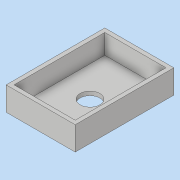
# Autodesk Inventor part: тело
Saved by Autodesk Inventor 2019 (Build 230136000, 136)
## iProperties
Created: 2019-09-06
Part Number: тело
Material: Типовые
Document SubType Name: Modeling
Designer: Iliga
Density: 1 g/cm^3
Appearance: По умолчанию
Mass: 236.83 g
Surface Area: 2382.33 cm^2
Volume: 236.83 cm^3
Author: Iliga
Autodesk Inventor part; units mm, degrees
ref_plane "РабПлоскость1" through (0, -35, 0) normal (0, 1, 0) x (-1, 0, 0)
ref_plane "РабПлоскость25" through (100, -155, 0) normal (-1, 0, 0) x (0, 0, 1)
ref_plane "РабПлоскость26" through (84, -165, -19) normal (-1, 0, 0) x (0, 0, 1)
sketch "Эскиз130" plane through (0, 0, 0) normal (0, 1, 0) x (-1, 0, 0)
  line L0 (-17.5, 25) -> (17.5, 25)
  line L1 (17.5, 25) -> (17.5, -25)
  line L2 (17.5, -25) -> (-17.5, -25)
  line L3 (-17.5, -25) -> (-17.5, 25)
  line L4 (-17.5, 25) -> (17.5, -25) construction
  line L5 (17.5, 25) -> (-17.5, -25) construction
  point P0 (0, 0)
  dimension "d710" = 50
  dimension "d711" = 35
  constraints: 12 end point, 2 midpoint, 2 parallel, 1 horizontal, 1 perpendicular
  measures "d710" distance of L0.end L1.end
  measures "d711" distance of L1.end L2.end
extrude "Выдавливание115" add sketch "Эскиз130" along normal blind 2
sketch "Эскиз131" plane through (0, 2, 0) normal (0, 1, 0) x (1, 0, 0)
  line L0 (15.5, -23) -> (-15.5, -23)
  line L1 (-15.5, -23) -> (-15.5, 23)
  line L2 (-15.5, 23) -> (15.5, 23)
  line L3 (15.5, 23) -> (15.5, -23)
  line L4 (15.5, -23) -> (-15.5, 23) construction
  line L5 (-15.5, -23) -> (15.5, 23) construction
  line L6 (-17.5, 25) -> (-17.5, -25) projected
  line L7 (17.5, 25) -> (-17.5, 25) projected
  line L8 (-17.5, -25) -> (17.5, -25) projected
  line L9 (17.5, -25) -> (17.5, 25) projected
  line L10 (-17.5, -25) -> (17.5, -25) projected
  line L11 (17.5, -25) -> (17.5, 25) projected
  line L12 (17.5, 25) -> (-17.5, 25) projected
  line L13 (-17.5, 25) -> (-17.5, -25) projected
  point P0 (0, 0)
  dimension "d714" = 2
  dimension "d715" = 2
  constraints: 12 end point, 2 midpoint, 2 parallel, 1 horizontal, 1 perpendicular
  measures "d714" distance between parallel lines of L1 L6
  measures "d715" distance between parallel lines of L7 L2
extrude "Выдавливание116" add sketch "Эскиз131" along normal blind 10
sketch "Эскиз132" plane through (0, 2, 0) normal (0, 1, 0) x (1, 0, 0)
  circle A0 centre (0, 0) radius 5
  dimension "d718" = 10
  dimension "d12" = 100
  dimension "d14" = 17
  dimension "d26" = 5
  constraints: 1 centre point, 1 coincident
  measures "d718" diameter of A0
extrude "Выдавливание117" cut sketch "Эскиз132" against normal blind 10
sketch "Эскиз6" plane through (0, -35, -85) normal (0, -1, 0) x (1, 0, 0)
  arc A0 (29.3991, 164.4544) -> (0, 170) centre (-5, 62.7941) ccw projected
  line L0 (0, 170) -> (0, 0) projected
  arc A1 (0, 0) -> (29.3991, 5.5456) centre (-5, 107.2059) ccw projected
  arc A2 (29.3991, 5.5456) -> (100, 85) centre (-5, 107.2059) ccw projected
  arc A3 (100, 85) -> (29.3991, 164.4544) centre (-5, 62.7941) ccw projected
  point P0 (0, 85)
  constraints: 4 end point, 1 horizontal, 1 point on circle, 1 vertical
sketch "Эскиз114" plane through (2, -165, 82.8837) normal (1, 0, 0) x (0, 0, -1)
  circle A0 centre (120.1897, 5) radius 1
  line L0 (-2.1163, 0) -> (167.8837, 0) construction
  line L1 (82.8837, 0) -> (82.8837, 60.2174) construction
  circle A1 centre (45.5777, 5) radius 1
  point P0 (82.8837, 165)
  dimension "d609" = 2
  dimension "d610" = 37.306
  dimension "d611" = 5
  constraints: 2 centre point, 2 end point, 1 midpoint, 1 symmetric about line, 1 vertical, 1 other
  measures "d609" diameter of A0
  measures "d610" distance from line of L1 A0.centre
  measures "d611" distance from line of L0 A0.centre
sketch "Эскиз115" plane through (2, -165, 82.8837) normal (1, 0, 0) x (0, 0, -1)
  line L0 (167.7717, 0) -> (0, 0) construction
  line L1 (82.8837, 130) -> (82.8837, 0) construction
  line L2 (63.8837, 0) -> (101.8837, 0)
  line L3 (101.8837, 0) -> (101.8837, 20)
  line L4 (101.8837, 20) -> (63.8837, 20)
  line L5 (63.8837, 20) -> (63.8837, 0)
  line L6 (65.8837, 2) -> (99.8837, 2)
  line L7 (99.8837, 2) -> (99.8837, 18)
  line L8 (99.8837, 18) -> (65.8837, 18)
  line L9 (65.8837, 18) -> (65.8837, 2)
  line L10 (65.8837, 2) -> (99.8837, 18) construction
  line L11 (99.8837, 2) -> (65.8837, 18) construction
  point P0 (82.8837, 165)
  point P1 (145.8837, 0)
  point P2 (82.8837, 20)
  point P3 (82.8837, 10)
  dimension "d614" = 38
  dimension "d615" = 20
  dimension "d616" = 2
  dimension "d617" = 2
  dimension "d618" = 2
  constraints: 20 end point, 4 parallel, 3 midpoint, 3 point on line, 2 horizontal, 2 perpendicular
  measures "d614" distance between parallel lines of L5 L3
  measures "d615" distance between parallel lines of L4 L0
  measures "d616" distance between parallel lines of L0 L6
  measures "d617" distance between parallel lines of L3 L7
  measures "d618" distance between parallel lines of L4 L8
sketch "Эскиз116" plane through (0, -165, -85) normal (0, -1, 0) x (1, 0, 0)
  arc A0 (91.9272, 104) -> (2, 167.8837) centre (-5, 62.7941) ccw construction
  arc A1 (97.9549, 85) -> (92.7533, 102) centre (-5, 62.7941) ccw construction
  arc A2 (97.9549, 85) -> (91.9272, 104) centre (-5, 62.7941) ccw construction
  arc A3 (91.9272, 66) -> (97.9549, 85) centre (-5, 107.206) ccw
  line L0 (2, 66) -> (100.2736, 66) construction
  arc A4 (100.2736, 66) -> (97.9549, 85) centre (-5, 62.7941) ccw projected
  line L1 (91.9272, 66) -> (100.2736, 66)
  point P0 (0, 85)
  point P1 (36.5, 159.5958)
  dimension "d621" = 22.206
  constraints: 2 end point, 2 point on circle, 1 centre point, 1 collinear, 1 point on line, 1 vertical alignment
  measures "d621" vertical distance of A3.centre point (0, 85)
sketch "Эскиз117" plane through (2, -165, 82.8837) normal (1, 0, 0) x (0, 0, -1)
  line L0 (101.8837, 20) -> (101.8837, 0) projected
  line L1 (63.8837, 20) -> (101.8837, 20) projected
  line L2 (63.8837, 0) -> (63.8837, 20) projected
  line L3 (63.8837, 0) -> (101.8837, 0)
  point P0 (82.8837, 165)
  constraints: 2 end point, 1 horizontal
sketch "Эскиз118" plane through (0, -165, -85) normal (0, -1, 0) x (1, 0, 0)
  line L0 (2, 66) -> (2, 104) projected
  line L1 (2, 66) -> (91.9272, 66) projected
  arc A0 (91.9272, 66) -> (97.9549, 85) centre (-5, 107.206) ccw projected
  line L2 (97.9549, 85) -> (100, 85) projected
  arc A1 (100, 85) -> (94.0968, 104) centre (-5, 62.7941) ccw projected
  line L3 (2, 104) -> (94.0968, 104) projected
  line L4 (2, 104) -> (4, 104)
  line L5 (4, 104) -> (4, 66)
  line L6 (4, 66) -> (2, 66)
  line L7 (2, 66) -> (2, 104)
  point P0 (0, 85)
  dimension "d626" = 2
  constraints: 8 end point, 2 parallel, 1 horizontal, 1 perpendicular, 1 point on line
  measures "d626" distance between parallel lines of L5 L0
sketch "Эскиз119" plane through (0, -165, -85) normal (0, -1, 0) x (1, 0, 0)
  arc A0 (100, 85) -> (94.0968, 104) centre (-5, 62.7941) ccw construction
  line L0 (4, 104) -> (4, 66) construction
  line L1 (4, 85) -> (65.3021, 85) construction
  arc A1 (94.0968, 66) -> (100, 85) centre (-5, 107.2059) ccw
  arc A2 (91.9272, 66) -> (97.9549, 85) centre (-5, 107.206) ccw construction
  line L2 (100, 85) -> (97.9549, 85)
  line L3 (94.0968, 66) -> (91.9272, 66)
  arc A3 (91.9272, 66) -> (97.9549, 85) centre (-5, 107.206) ccw
  point P0 (0, 85)
  constraints: 6 end point, 4 point on circle, 2 centre point, 2 horizontal, 2 symmetric about line, 1 coincident, 1 midpoint, 1 parallel, 1 point on line, 1 other
sketch "Эскиз120" plane through (4, -147, 17) normal (0, -1, 0) x (1, 0, 0)
  line L0 (0, 0) -> (2, 0)
  line L1 (2, 0) -> (2, -34)
  line L2 (2, -34) -> (0, -34)
  line L3 (0, -34) -> (0, 0)
  point P0 (-4, -17)
  dimension "d631" = 2
  constraints: 8 end point, 2 parallel, 1 coincident, 1 horizontal, 1 perpendicular
  measures "d631" distance between parallel lines of L3 L1
sketch "Эскиз121" plane through (0, 0, 0) normal (1, 0, 0) x (0, 1, 0)
  line L0 (-145, -19) -> (-145, 19) construction
  line L1 (-165, -19) -> (-145, -19) construction
  line L2 (-165, 19) -> (-165, -19) construction
  line L3 (-145, 19) -> (-165, 19) construction
  line L4 (-158, -19) -> (-152, -19)
  line L5 (-152, -19) -> (-152, -25)
  line L6 (-152, -25) -> (-158, -25)
  line L7 (-158, -25) -> (-158, -19)
  circle A0 centre (-155, -22) radius 1
  line L8 (-158, 25) -> (-152, 25)
  line L9 (-152, 25) -> (-152, 19)
  line L10 (-152, 19) -> (-158, 19)
  line L11 (-158, 19) -> (-158, 25)
  circle A1 centre (-155, 22) radius 1
  line L12 (-155, 19) -> (-155, -19) construction
  point P0 (0, 0)
  dimension "d634" = 6
  dimension "d635" = 6
  dimension "d636" = 2
  dimension "d637" = 3
  dimension "d638" = 3
  dimension "d639" = 6
  dimension "d640" = 6
  dimension "d641" = 2
  dimension "d642" = 3
  dimension "d643" = 3
  constraints: 18 end point, 4 midpoint, 4 parallel, 2 centre point, 2 horizontal, 2 perpendicular
  measures "d634" distance of L5.end L6.end
  measures "d635" distance of L4.end L5.end
  measures "d636" diameter of A0
  measures "d637" distance from line of L6 A0.centre
  measures "d638" distance from line of L7 A0.centre
  measures "d639" distance of L9.end L10.end
  measures "d640" distance of L8.end L9.end
  measures "d641" diameter of A1
  measures "d642" distance from line of L10 A1.centre
  measures "d643" distance from line of L11 A1.centre
sketch "Эскиз122" plane through (0, -158, 19) normal (0, -1, 0) x (1, 0, 0)
  line L0 (0, 0) -> (0, 6) projected
  line L1 (0, 0) -> (4, 0) projected
  line L2 (6, 0) -> (4, 0) projected
  line L3 (6, 6) -> (6, 0) projected
  line L4 (0, 6) -> (6, 6) projected
  line L5 (0, -44) -> (0, -38) projected
  line L6 (0, -44) -> (6, -44) projected
  line L7 (6, -38) -> (6, -44) projected
  line L8 (4, -38) -> (6, -38) projected
  line L9 (0, -38) -> (4, -38) projected
  line L10 (0, 6) -> (4, 6)
  line L11 (4, 6) -> (4, -44)
  line L12 (4, -44) -> (0, -44)
  line L13 (0, -44) -> (0, 6)
  line L14 (0, -44) -> (6, -44) projected
  point P0 (0, -19)
  dimension "d646" = 4
  constraints: 8 end point, 2 parallel, 1 horizontal, 1 perpendicular, 1 point on line
  measures "d646" distance between parallel lines of L11 L13
sketch "Эскиз123" plane through (0, -165, -85) normal (0, -1, 0) x (1, 0, 0)
  line L0 (32, 66) -> (34, 66)
  line L1 (34, 66) -> (34, 63)
  line L2 (34, 63) -> (32, 63)
  line L3 (32, 63) -> (32, 66)
  line L4 (4, 104) -> (4, 66) projected
  line L5 (94.0968, 66) -> (4, 66) projected
  line L6 (32, 107) -> (34, 107)
  line L7 (34, 107) -> (34, 104)
  line L8 (34, 104) -> (32, 104)
  line L9 (32, 104) -> (32, 107)
  line L10 (4, 104) -> (94.0968, 104) projected
  line L11 (36.5, 107) -> (38.5, 107)
  line L12 (38.5, 107) -> (38.5, 104)
  line L13 (38.5, 104) -> (36.5, 104)
  line L14 (36.5, 104) -> (36.5, 107)
  line L15 (36.5, 66) -> (38.5, 66)
  line L16 (38.5, 66) -> (38.5, 63)
  line L17 (38.5, 63) -> (36.5, 63)
  line L18 (36.5, 63) -> (36.5, 66)
  point P0 (0, 85)
  dimension "d650" = 30
  dimension "d651" = 2
  dimension "d652" = 3
  dimension "d653" = 2
  dimension "d654" = 3
  dimension "d655" = 2
  dimension "d656" = 3
  dimension "d657" = 2
  dimension "d658" = 3
  dimension "d659" = 30
  dimension "d660" = 2.5
  dimension "d661" = 2.5
  constraints: 32 end point, 8 parallel, 4 horizontal, 4 perpendicular, 4 point on line
  measures "d650" distance between parallel lines of L4 L1
  measures "d651" distance between parallel lines of L1 L3
  measures "d652" distance of L0.end L1.end
  measures "d653" distance between parallel lines of L7 L9
  measures "d654" distance of L6.end L7.end
  measures "d655" distance between parallel lines of L12 L14
  measures "d656" distance of L11.end L12.end
  measures "d657" distance between parallel lines of L16 L18
  measures "d658" distance of L15.end L16.end
  measures "d659" distance between parallel lines of L4 L7
  measures "d660" distance between parallel lines of L14 L7
  measures "d661" distance between parallel lines of L18 L1
sketch "Эскиз124" plane through (36.5, -145, -19) normal (0, 0, 1) x (1, 0, 0)
  line L0 (0, 0) -> (2, 0) projected
  line L1 (2, 0) -> (2, 2) projected
  line L2 (0, 2) -> (2, 2) projected
  line L3 (0, 0) -> (0, 2) projected
  line L4 (-4.5, 0) -> (-2.5, 0) projected
  line L5 (-2.5, 0) -> (-2.5, 2) projected
  line L6 (-4.5, 2) -> (-2.5, 2) projected
  line L7 (-4.5, 0) -> (-4.5, 2) projected
  point P0 (-36.5, 145)
  dimension "d667" = 2
  dimension "d668" = 9.5
  dimension "d669" = 10
  constraints: 2 centre point, 2 end point, 1 symmetric about line, 1 vertical, 1 other
sketch "Эскиз126" plane through (0, -165, -85) normal (0, -1, 0) x (1, 0, 0)
  circle A0 centre (16, 79) radius 1
  circle A1 centre (16, 91) radius 1
  line L0 (4, 104) -> (4, 66) projected
  line L1 (4, 85) -> (100.0263, 85) construction
  circle A2 centre (31, 79) radius 1
  circle A3 centre (31, 91) radius 1
  circle A4 centre (71, 75) radius 1
  circle A5 centre (71, 95) radius 1
  point P0 (0, 85)
  dimension "d674" = 2
  dimension "d675" = 2
  dimension "d676" = 12
  dimension "d677" = 12
  dimension "d678" = 6
  dimension "d679" = 2
  dimension "d680" = 2
  dimension "d681" = 12
  dimension "d683" = 27
  dimension "d684" = 6
  dimension "d685" = 2
  dimension "d686" = 2
  dimension "d689" = 67
  dimension "d690" = 10
  dimension "d697" = 20
  constraints: 6 centre point, 3 vertical alignment, 2 end point, 1 horizontal, 1 midpoint
  measures "d674" diameter of A0
  measures "d675" diameter of A1
  measures "d676" distance from line of L0 A0.centre
  measures "d677" distance of A1.centre A0.centre
  measures "d678" distance from line of L1 A0.centre
  measures "d679" diameter of A2
  measures "d680" diameter of A3
  measures "d681" distance of A3.centre A2.centre
  measures "d683" distance from line of L0 A2.centre
  measures "d684" distance from line of L1 A2.centre
  measures "d685" diameter of A4
  measures "d686" diameter of A5
  measures "d689" distance from line of L0 A4.centre
  measures "d690" distance from line of L1 A4.centre
  measures "d697" distance of A5.centre A4.centre
sketch "Эскиз127" plane through (0, -165, -85) normal (0, -1, 0) x (1, 0, 0)
  circle A0 centre (71, 75) radius 1 construction
  circle A1 centre (31, 79) radius 1 construction
  circle A2 centre (16, 79) radius 1 construction
  circle A3 centre (16, 91) radius 1 construction
  circle A4 centre (31, 91) radius 1 construction
  circle A5 centre (71, 95) radius 1 construction
  arc A6 (32, 64) -> (34, 64) centre (33, 64) ccw construction
  line L0 (34, 64) -> (34, 66) construction
  line L1 (36.5, 66) -> (34, 66) construction
  line L2 (36.5, 66) -> (36.5, 64) construction
  arc A7 (36.5, 64) -> (38.5, 64) centre (37.5, 64) ccw construction
  line L3 (38.5, 64) -> (38.5, 66) construction
  line L4 (94.0968, 66) -> (38.5, 66) construction
  arc A8 (94.0968, 66) -> (100, 85) centre (-5, 107.2059) ccw projected
  arc A9 (100, 85) -> (94.0968, 104) centre (-5, 62.7941) ccw projected
  line L5 (38.5, 104) -> (94.0968, 104) construction
  line L6 (38.5, 104) -> (38.5, 106) construction
  arc A10 (38.5, 106) -> (36.5, 106) centre (37.5, 106) ccw construction
  line L7 (36.5, 106) -> (36.5, 104) construction
  line L8 (34, 104) -> (36.5, 104) construction
  line L9 (34, 104) -> (34, 106) construction
  arc A11 (34, 106) -> (32, 106) centre (33, 106) ccw construction
  line L10 (32, 106) -> (32, 104) construction
  line L11 (4, 104) -> (32, 104) construction
  line L12 (4, 104) -> (4, 66) construction
  line L13 (32, 66) -> (4, 66) construction
  line L14 (32, 66) -> (32, 64) construction
  line L15 (4, 85) -> (100, 85) construction
  line L16 (4, 84) -> (99.7835, 84)
  line L17 (4, 86) -> (99.7835, 86)
  line L18 (4, 86) -> (4, 84)
  point P0 (0, 85)
  dimension "d693" = 2
  dimension "d694" = 1
  constraints: 8 end point, 2 parallel, 2 point on circle, 2 point on line, 1 horizontal, 1 midpoint, 1 vertical
  measures "d693" distance between parallel lines of L17 L16
  measures "d694" distance between parallel lines of L15 L16
sketch "Эскиз128" plane through (84, -165, -19) normal (-1, 0, 0) x (0, 0, 1)
  line L0 (-7, 0) -> (46, 0)
  line L1 (46, 0) -> (46, 24)
  line L2 (46, 24) -> (-7, 24)
  line L3 (-7, 24) -> (-7, 0)
  point P0 (19, 165)
  point P1 (0, 0)
  dimension "d699" = 53
  dimension "d700" = 24
  dimension "d701" = 7
  constraints: 8 end point, 2 parallel, 1 horizontal, 1 perpendicular, 1 point on line
  measures "d699" distance of L1.end L2.end
  measures "d700" distance of L2.end L0.start
  measures "d701" distance from line of point (0, 0) L3
sketch "Эскиз129" plane through (38.5, -145, 19) normal (0, 1, 0) x (1, 0, 0)
  arc A0 (45.5, 48) -> (45.5, -10) centre (79.9093, 19) ccw
  line L0 (45.5, 48) -> (45.5, -10)
  line L1 (45.5, 0) -> (45.5, 38) projected
  line L2 (0, 0) -> (45.5, 0) projected
  point P0 (-38.5, 19)
  dimension "d707" = 10
  dimension "d708" = 10
  dimension "d709" = 45
  dimension "d10" = 170
  dimension "d15" = 4
  dimension "d16" = 35
  dimension "d97" = 2
  constraints: 10 end point, 3 point on circle, 2 horizontal, 2 vertical alignment, 1 centre point, 1 horizontal alignment, 1 perpendicular, 1 vertical
  measures "d10" distance of L0.start L0.end
  measures "d15" distance of point (0, 0) A0.centre
